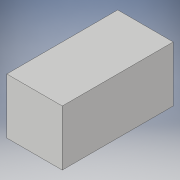
# Autodesk Inventor part: 1x2 beam
Saved by Autodesk Inventor 2019 (Build 230136000, 136)
## iProperties
Created: 2020-03-28
Part Number: 1x2 beam
Material: Generic
Document SubType Name: Modeling
Designer: q
Density: 1 g/cm^3
Appearance: Default
Author: q
Autodesk Inventor part; units mm, degrees
ref_plane "YZ Plane" through (0, 0, 0) normal (1, 0, 0) x (0, 1, 0)
ref_plane "XZ Plane" through (0, 0, 0) normal (0, 1, 0) x (-1, 0, 0)
ref_plane "XY Plane" through (0, 0, 0) normal (0, 0, 1) x (1, 0, 0)
sketch "Sketch1" plane through (0, 0, 0) normal (1, 0, 0) x (0, 1, 0)
  line L0 (0, 0) -> (250, 0)
  line L1 (250, 0) -> (250, -500)
  line L2 (250, -500) -> (0, -500)
  line L3 (0, -500) -> (0, 0)
  dimension "d0" = 250
  dimension "d1" = 500
  constraints: 8 end point, 2 parallel, 1 horizontal, 1 perpendicular
  measures "d0" distance of L1.end L2.end
  measures "d1" distance of L0.end L1.end
extrude "Extrusion1" add sketch "Sketch1" along normal blind 250
body "Solid1"
